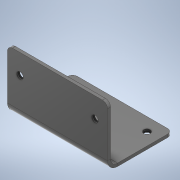
# Autodesk Inventor part: Clamp_Plate
Saved by Autodesk Inventor 2020 (Build 240168000, 168)
## iProperties
Created: 2021-07-08
Part Number: Clamp_Plate
Material: Steel, Carbon
Document SubType Name: Sheet Metal
Designer: Simon.Alvarez
Density: 7.85 g/cm^3
Sheet Metal Rule: Default_mm
Appearance: Semi-Polished
Author: Simon.Alvarez
Autodesk Inventor part; units mm, degrees
ref_plane "YZ Plane" through (0, 0, 0) normal (1, 0, 0) x (0, 1, 0)
ref_plane "XZ Plane" through (0, 0, 0) normal (0, 1, 0) x (-1, 0, 0)
ref_plane "XY Plane" through (0, 0, 0) normal (0, 0, 1) x (1, 0, 0)
sketch "Sketch1" plane through (0, 0, 0) normal (0, 0, 1) x (1, 0, 0)
  line L0 (-50, -30) -> (50, -30)
  line L1 (50, -30) -> (50, 30)
  line L2 (50, 30) -> (-50, 30)
  line L3 (-50, 30) -> (-50, -30)
  line L4 (-50, -30) -> (50, 30) construction
  line L5 (50, -30) -> (-50, 30) construction
  point P0 (0, 0)
  dimension "d0" = 60
  dimension "d1" = 100
  constraints: 12 end point, 2 midpoint, 2 parallel, 1 horizontal, 1 perpendicular
  measures "d0" distance of L2.end L0.start
  measures "d1" distance of L1.end L2.end
extrude "Extrusion1" add sketch "Sketch1" along normal blind 3
sketch "Sketch2" plane through (-50, -27, 3) normal (0, -1, 0) x (1, 0, 0)
  line L0 (100, 0) -> (0, 0)
  line L1 (0, 0) -> (0, -65)
  line L2 (0, -65) -> (100, -65)
  line L3 (100, -65) -> (100, 0)
  constraints: 6 end point, 1 horizontal, 1 perpendicular, 1 vertical
edge flange "Flange1" height 65 angle 90 thickness 3 bend radius 7 thickness toward (0, -1, 0) relief tear relief width 3 relief depth 1.5 edges at (0, -30, 0) wall of the first edge with corners at (50, -27, 3) (-50, -27, 3) (-50, -27, -62) (50, -27, -62)
bend "Bend1"
corner "Corner1"
sketch "Sketch3" plane through (0, 0, 3) normal (0, 0, 1) x (1, 0, 0)
  line L0 (50, 30) -> (-50, 30) projected
  point P0 (0, 0)
  point P1 (-37.5, 10)
  point P2 (37.5, 10)
  dimension "d15" = 20
  dimension "d16" = 37.5
  dimension "d17" = 75
  constraints: 1 horizontal alignment
  measures "d15" distance from line of point (-37.5, 10) L0
  measures "d16" horizontal distance of point (0, 0) point (-37.5, 10)
  measures "d17" distance of point (37.5, 10) point (-37.5, 10)
hole "Hole1" at (-37.5, 10, 3) at (37.5, 10, 3) direction (0, 0, -1) diameter 6.647 end through all thread size "M8x1.25" class "6H" standard "ANSI Metric M Profile"
sketch "Sketch4" plane through (-50, -27, -62) normal (0, 1, 0) x (1, 0, 0)
  line L0 (0, -65) -> (100, -65) projected
  line L1 (50, -65) -> (50, 0) construction
  line L2 (100, 0) -> (0, 0) projected
  point P0 (50, -62)
  point P1 (87.5, -13)
  point P2 (12.5, -13)
  dimension "d26" = 37.5
  dimension "d27" = 75
  dimension "d36" = 52
  constraints: 2 end point, 2 midpoint, 1 horizontal alignment
  measures "d26" distance from line of L1 point (87.5, -13)
  measures "d27" distance of point (12.5, -13) point (87.5, -13)
  measures "d36" distance from line of L0 point (87.5, -13)
hole "Hole2" at (37.5, -27, -49) at (-37.5, -27, -49) direction (0, -1, 0) diameter 6.647 end through all thread size "M8x1.25" class "6H" standard "ANSI Metric M Profile"
fillet "Fillet1" radius 5 4 edges at (-50, 30, 1.5) (50, 30, 1.5) (-50, -28.5, -62) (50, -28.5, -62)
equation "\"d1\" = Width"
equation "\"d4\" = Thickness"
equation "\"d5\" = BendReliefWidth"
equation "\"d6\" = BendReliefDepth"
equation "\"d7\" = MinimumRemnant"
equation "\"d8\" = TransitionRadius"
equation "\"d12\" = CornerReliefSize"
equation "\"d13\" = GapSize"
equation "\"d14\" = JacobiRadiusSize"
equation "\"d16\" = 0.5 * Bolt_Width"
equation "\"d17\" = Bolt_Width"
equation "\"d26\" = 0.5 * Bolt_Width"
equation "\"d27\" = Bolt_Width"
equation "\"BendRadius\" = Thickness"
equation "\"BendReliefWidth\" = Thickness"
equation "\"BendReliefDepth\" = 0.5 * Thickness"
equation "\"CornerReliefSize\" = 4 * Thickness"
equation "\"MinimumRemnant\" = 2 * Thickness"
equation "\"TransitionRadius\" = BendRadius"
equation "\"JacobiRadiusSize\" = BendRadius"
equation "\"GapSize\" = Thickness"
equation "\"Width\" = 100"
equation "\"Thickness\" = 3"
equation "\"Bolt_Width\" = 75"
body "Solid1"
